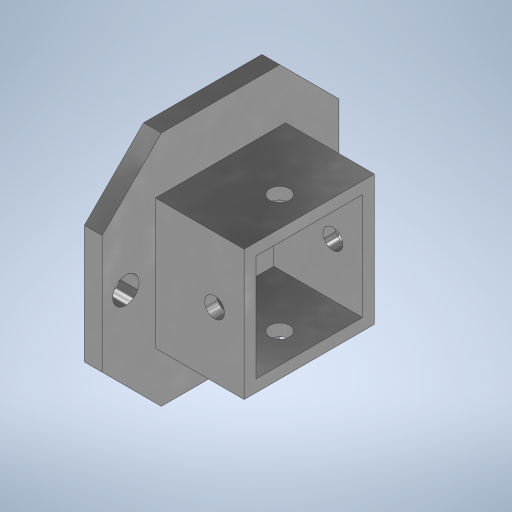
# Autodesk Inventor part: square_ber_holder
Saved by Autodesk Inventor 2024 (Build 280153000, 153)
## iProperties
Created: 2025-01-22
Part Number: square_ber_holder
Material: ABS プラスチック
Document SubType Name: Modeling
Designer: 1412z
Density: 1.06 g/cm^3
Appearance: オニキス - 黒
Author: 1412z
Autodesk Inventor part; units mm, degrees
ref_plane "YZ Plane" through (0, 0, 0) normal (1, 0, 0) x (0, 1, 0)
ref_plane "XZ Plane" through (0, 0, 0) normal (0, 1, 0) x (-1, 0, 0)
ref_plane "XY Plane" through (0, 0, 0) normal (0, 0, 1) x (1, 0, 0)
sketch "スケッチ1" plane through (0, 0, 0) normal (1, 0, 0) x (0, 1, 0)
  line L0 (9, -9) -> (-9, -9)
  line L1 (-9, -9) -> (-9, 9)
  line L2 (-9, 9) -> (9, 9)
  line L3 (9, 9) -> (9, -9)
  line L4 (9, -9) -> (-9, 9) construction
  line L5 (-9, -9) -> (9, 9) construction
  line L6 (11, -11) -> (-11, -11)
  line L7 (-11, -11) -> (-11, 11)
  line L8 (-11, 11) -> (11, 11)
  line L9 (11, 11) -> (11, -11)
  line L10 (11, -11) -> (-11, 11) construction
  line L11 (-11, -11) -> (11, 11) construction
  point P0 (0, 0)
  dimension "d0" = 18
  dimension "d1" = 18
  dimension "d2" = 22
  dimension "d3" = 22
  constraints: 24 end point, 4 midpoint, 4 parallel, 2 horizontal, 2 perpendicular
  measures "d0" distance of L1.end L2.end
  measures "d1" distance of L0.end L1.end
  measures "d2" distance of L7.end L8.end
  measures "d3" distance of L6.end L7.end
extrude "押し出し1" add sketch "スケッチ1" along normal blind 15
sketch "スケッチ2" plane through (0, -11, 11) normal (0, 0, 1) x (1, 0, 0)
  circle A0 centre (10, 11) radius 1.7
  point P0 (0, 11)
  dimension "d6" = 3.4
  constraints: 1 centre point
  measures "d6" diameter of A0
extrude "押し出し2" cut sketch "スケッチ2" against normal blind 30
sketch "スケッチ3" plane through (0, 11, 11) normal (0, 1, 0) x (1, 0, 0)
  circle A0 centre (10, 11) radius 1.7
  point P0 (0, 11)
  dimension "d9" = 3.4
  constraints: 1 centre point
  measures "d9" diameter of A0
extrude "押し出し3" cut sketch "スケッチ3" against normal blind 30
sketch "スケッチ4" plane through (0, 0, 0) normal (-1, 0, 0) x (0, 0, 1)
  line L0 (20, -20) -> (-20, -20)
  line L1 (-20, -20) -> (-20, 20)
  line L2 (-20, 20) -> (20, 20)
  line L3 (20, 20) -> (20, -20)
  line L4 (20, -20) -> (-20, 20) construction
  line L5 (-20, -20) -> (20, 20) construction
  point P0 (0, 0)
  dimension "d12" = 40
  dimension "d13" = 40
  constraints: 12 end point, 2 midpoint, 2 parallel, 1 horizontal, 1 perpendicular
  measures "d12" distance of L1.end L2.end
  measures "d13" distance of L0.end L1.end
extrude "押し出し4" add sketch "スケッチ4" along normal blind 3
sketch "スケッチ5" plane through (-3, 0, 0) normal (-1, 0, 0) x (0, 0, 1)
  circle A0 centre (16, 0) radius 2.25
  circle A1 centre (-16, 0) radius 2.25
  point P0 (0, 0)
  dimension "d16" = 4.5
  dimension "d17" = 4.5
  constraints: 2 centre point
  measures "d16" diameter of A0
  measures "d17" diameter of A1
extrude "押し出し5" cut sketch "スケッチ5" against normal blind 3
sketch "スケッチ6" plane through (-3, 0, 0) normal (-1, 0, 0) x (0, 0, 1)
  line L0 (20, 20) -> (-20, 20) projected
  line L1 (10, 20) -> (20, 10)
  line L2 (20, -20) -> (20, 20) projected
  line L3 (10, 20) -> (24.1421, 20) construction
  line L4 (20, 10) -> (20, 20)
  line L5 (20, 20) -> (10, 20)
  line L6 (-20, -20) -> (20, -20) projected
  line L7 (20, -20) -> (10, -20)
  line L8 (10, -20) -> (20, -10)
  line L9 (20, -10) -> (20, -20)
  line L10 (-20, 20) -> (-20, -20) projected
  line L11 (-20, -20) -> (-10, -20)
  line L12 (-10, -20) -> (-20, -10)
  line L13 (-20, -10) -> (-20, -20)
  line L14 (-20, 20) -> (-10, 20)
  line L15 (-10, 20) -> (-20, 10)
  line L16 (-20, 10) -> (-20, 20)
  point P0 (0, 0)
  dimension "d20" = 45
  dimension "d21" = 10
  dimension "d22" = 45
  dimension "d23" = 10
  dimension "d24" = 45
  dimension "d25" = 10
  dimension "d26" = 45
  constraints: 26 end point, 9 point on line, 4 perpendicular, 1 equal length, 1 horizontal, 1 vertical
  measures "d20" angle of L1 L3
  measures "d21" distance of L2.start L7.end
  measures "d22" angle of L7 L8
  measures "d23" distance of L6.start L11.end
  measures "d24" angle of L12 L11
  measures "d25" distance of L14.start L14.end
  measures "d26" angle of L14 L15
extrude "押し出し6" cut sketch "スケッチ6" against normal blind 3 contours L2 L1 L0 | L15 L10 L0 | L2 L6 L8 | L12 L6 L10
